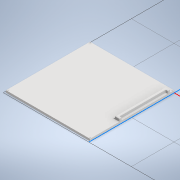
# Autodesk Inventor part: box_bottom
Saved by Autodesk Inventor 2020 (Build 240168000, 168)
## iProperties
Created: 2020-02-22
Part Number: box_bottom
Material: Generic
Document SubType Name: Modeling
Designer: Luka
Density: 1 g/cm^3
Appearance: Default
Author: Luka
Autodesk Inventor part; units mm, degrees
ref_plane "YZ Plane" through (0, 0, 0) normal (1, 0, 0) x (0, 1, 0)
sketch "Sketch1" plane through (0, 0, 0) normal (0, 1, 0) x (-1, 0, 0)
  line L0 (200, 200) -> (0, 200)
  line L1 (0, 200) -> (0, 0)
  line L2 (0, 0) -> (200, 0)
  line L3 (200, 0) -> (200, 200)
  dimension "d0" = 200
  dimension "d1" = 200
  constraints: 8 end point, 2 parallel, 1 horizontal, 1 perpendicular
  measures "d0" distance of L2.end L1.end
  measures "d1" distance of L1.end L0.end
extrude "Extrusion1" add sketch "Sketch1" along normal blind 200
shell "Shell1" thickness 5 removed faces 1 at (-66.6667, 200, 133.3333)
sketch "Sketch2" plane through (-200, 0, 200) normal (0, 0, 1) x (1, 0, 0)
  line L0 (155, 160) -> (158.5, 160)
  line L1 (158.5, 160) -> (158.5, 130)
  line L2 (158.5, 130) -> (155, 130)
  line L3 (155, 130) -> (155, 160)
  line L4 (0, 0) -> (0, 200) projected
  line L5 (200, 0) -> (200, 200) projected
  line L6 (0, 200) -> (200, 200) projected
  line L7 (120, 160) -> (40, 160)
  line L8 (40, 160) -> (40, 125)
  line L9 (40, 125) -> (120, 125)
  line L10 (120, 125) -> (120, 160)
  line L11 (40, 115) -> (120, 115)
  line L12 (120, 115) -> (120, 35)
  line L13 (120, 35) -> (40, 35)
  line L14 (40, 35) -> (40, 115)
  line L15 (69, 25) -> (91, 25)
  line L16 (91, 25) -> (91, 21)
  line L17 (91, 21) -> (69, 21)
  line L18 (69, 21) -> (69, 25)
  line L19 (44, 155) -> (116, 155)
  line L20 (116, 155) -> (116, 130)
  line L21 (116, 130) -> (44, 130)
  line L22 (44, 130) -> (44, 155)
  circle A0 centre (40, 160) radius 5
  circle A1 centre (120, 160) radius 5
  circle A2 centre (120, 125) radius 5
  circle A3 centre (40, 125) radius 5
  line L23 (69, 25) -> (91, 25)
  line L24 (91, 25) -> (91, 35)
  line L25 (91, 35) -> (69, 35)
  line L26 (69, 35) -> (69, 25)
  point P0 (120, 155)
  point P1 (115, 160)
  point P2 (115, 125)
  point P3 (120, 130)
  point P4 (40, 130)
  point P5 (45, 125)
  point P6 (45, 160)
  point P7 (40, 155)
  point P8 (69, 35)
  point P9 (91, 25)
  dimension "COINw" = 3.5
  dimension "COINh" = 30
  dimension "d7" = 155
  dimension "d8" = 41.5
  dimension "d12" = 40
  dimension "d13" = 40
  dimension "LCDw" = 80
  dimension "LCDh" = 35
  dimension "d19" = 22
  dimension "d20" = 4
  dimension "d22" = 29
  dimension "d23" = 10
  dimension "d24" = 10
  dimension "d27" = 72
  dimension "d28" = 25
  dimension "d29" = 4
  dimension "d30" = 4
  dimension "d31" = 5
  dimension "d32" = 5
  dimension "d33" = 10
  dimension "d34" = 10
  dimension "d35" = 10
  constraints: 48 end point, 12 parallel, 7 perpendicular, 6 horizontal, 4 centre point, 4 coincident, 4 collinear, 1 point on line
  measures "COINw" distance of L1.end L2.end
  measures "COINh" distance of L0.end L1.end
  measures "d7" distance between parallel lines of L4 L3
  measures "d8" distance between parallel lines of L5 L1
  measures "d12" distance between parallel lines of L6 L0
  measures "d13" distance between parallel lines of L8 L4
  measures "LCDw" distance between parallel lines of L10 L8
  measures "LCDh" distance between parallel lines of L9 L7
  measures "d19" distance of L15.start L15.end
  measures "d20" distance of L15.end L16.end
  measures "d22" distance from line of L13.end L18
  measures "d23" distance between parallel lines of L15 L13
  measures "d24" distance between parallel lines of L11 L9
  measures "d27" distance of L20.end L21.end
  measures "d28" distance of L19.end L20.end
  measures "d29" distance between parallel lines of L8 L22
  measures "d30" distance between parallel lines of L10 L20
  measures "d31" distance between parallel lines of L7 L19
  measures "d32" distance between parallel lines of L9 L21
  measures "d33" diameter of A0
  measures "d34" diameter of A2
  measures "d35" diameter of A3
extrude "Extrusion2" cut sketch "Sketch2" along normal mid plane 10 contours L0 L1 L2 L3 | L15 L16 L17 L18 | L19 L20 L21 L22
fillet "Fillet1" radius 2 4 edges at (-195, 200, 100) (-100, 200, 5) (-5, 200, 100) (-100, 200, 195)
sketch "Sketch3" plane through (0, 0, 200) normal (1, 0, 0) x (0, 0, -1)
  line L0 (0, 0) -> (0, 200) projected
  line L1 (0, 80) -> (200, 80)
  line L2 (0, 0) -> (200, 0) projected
  line L3 (195, 5) -> (195, 198) projected
  line L4 (195, 80) -> (195, 0)
  line L5 (95, 80) -> (95, 0)
  line L6 (200, 0) -> (0, 0) projected
  line L7 (5, 5) -> (195, 5) projected
  line L8 (95, 5) -> (195, 5)
  dimension "d16" = 80
  dimension "d44" = 100
  constraints: 8 end point, 8 point on line, 2 perpendicular, 1 collinear, 1 horizontal
  measures "d16" distance between parallel lines of L2 L1
  measures "d44" distance between parallel lines of L3 L5
extrude "Extrusion3" cut sketch "Sketch2" against normal blind 2 contours A0 L8 L7 | L7 L8 A0 | L7 A1 L10 A2 L9 A3 L8 A0 | A1 L10 L7 | L7 L10 A1 | A3 L9 L8 | L8 L9 A3 | A2 L9 L10 | L10 L9 A2 | L11 L12 L13 L14 | L13 L24 L15 L26 | L19 L20 L21 L22
hole "Hole1" at (-160, 160, 200) at (-80, 160, 200) at (-80, 125, 200) at (-160, 125, 200) direction (0, 0, -1) diameter 3.5 depth 5
fillet "Fillet2" radius 3 5 edges at (-160, 75, 198) (-80, 75, 198) (-94.5, 35, 198) (-145.5, 35, 198) (-120, 115, 198)
extrude "Extrusion4" cut sketch "Sketch3" against normal blind 5 contours L1 L3 L7 L5
sketch "Sketch4" plane through (0, 5, 105) normal (0, 0, -1) x (-1, 0, 0)
  circle A0 centre (2.5, 73.5) radius 2.5
  line L0 (0, 0) -> (0, 75) projected
  line L1 (5, 75) -> (5, 0) projected
  circle A1 centre (2.5, 73.5) radius 1
  line L2 (0, 75) -> (5, 75) projected
  line L3 (2.5, 76) -> (2.5, 73.5)
  line L4 (2.5, 73.5) -> (2.5, 71)
  line L5 (2.5, 71) -> (5, 71)
  line L6 (2.5, 76) -> (5, 76)
  line L7 (0, 75) -> (5, 75) projected
  line L8 (5, 76) -> (5, 75)
  point P0 (0, -5)
  point P1 (4.5, 75)
  point P2 (0.5, 75)
  dimension "d47" = 2
  dimension "d48" = 1.5
  constraints: 10 end point, 4 tangent, 2 centre point, 2 perpendicular, 2 point on circle, 2 point on line, 1 coincident, 1 parallel, 1 vertical
  measures "d47" diameter of A1
  measures "d48" distance from line of A0.centre L2
extrude "Extrusion5" add sketch "Sketch4" along normal blind 80 contours L4 A1 L3 L2 A0 | A0 L2 L3 A1 L4
extrude "Extrusion6" cut sketch "Sketch4" along normal blind 60 contours L4 A1 L3 L2 A0 | A0 L2 L3 A1 L4
extrude "Extrusion7" add sketch "Sketch4" along normal blind 40 contours L4 A1 L3 L2 A0 | A0 L2 L3 A1 L4
extrude "Extrusion8" cut sketch "Sketch4" along normal blind 20 contours L4 A1 L3 L2 A0 | A0 L2 L3 A1 L4
fillet "Fillet3" radius 3 2 edges at (-0.5, 80, 75) (-0.5, 80, 35)
fillet "Fillet4" radius 4 2 edges at (-4.5, 80, 75) (-4.5, 80, 35)
extrude "Extrusion9" cut sketch "Sketch4" against normal blind 40 contours L4 L3 A1 | A1 L3 L4
ref_plane "Work Plane1" through (0, 5, 120) normal (0, 0, -1) x (-1, 0, 0)
sketch "Sketch5" plane through (0, 5, 120) normal (0, 0, -1) x (-1, 0, 0)
  circle A0 centre (2.5, 73.5) radius 2.5 projected
  circle A1 centre (2.5, 73.5) radius 1 projected
  line L0 (2.5, 71) -> (5, 71) projected
  line L1 (5, 75) -> (5, 0) projected
  line L2 (5, 71) -> (5, 75)
  line L3 (5, 75) -> (5, 76)
  line L4 (5, 75) -> (5, 193) projected
  line L5 (2.5, 76) -> (5, 76)
  line L6 (2.5, 76) -> (2.5, 71)
  point P0 (0, -5)
  constraints: 8 end point, 1 collinear, 1 point on circle, 1 point on line, 1 tangent, 1 vertical
extrude "Extrusion10" cut sketch "Sketch5" against normal blind 25 contours A0 L6 A1 | L1 L0 A0 | A0 L5 L3 L1 | A1 L6 picked at (4.2027, 74.5258) picked at (3.0499, 73.7078)
ref_plane "Work Plane4" through (-195, 5, 5) normal (0, 1, 0) x (1, 0, 0)
split "Split1" plane through (-195, 5, 5) removes the side toward (0, 1, 0)
sketch "Sketch6" plane through (-200, 5, 0) normal (0, 1, 0) x (1, 0, 0)
  line L0 (200, 0) -> (200, -200) projected
  line L1 (200, -10) -> (195, -10)
  line L2 (195, -10) -> (195, -15)
  line L3 (195, -15) -> (200, -15)
  line L4 (0, 0) -> (200, 0) projected
  line L5 (200, -125) -> (195, -125)
  line L6 (195, -125) -> (195, -130)
  line L7 (195, -130) -> (200, -130)
  line L8 (195, -130) -> (190, -130)
  line L9 (190, -130) -> (190, -10)
  line L10 (190, -10) -> (195, -10)
  line L11 (195, -10) -> (195, -130)
  dimension "d66" = 10
  dimension "d67" = 5
  dimension "d68" = 5
  dimension "d71" = 5
  dimension "d72" = 110
  dimension "d73" = 5
  dimension "d89" = 5
  constraints: 20 end point, 5 perpendicular, 4 point on line, 3 horizontal, 2 parallel, 1 collinear
  measures "d66" distance between parallel lines of L4 L1
  measures "d67" distance between parallel lines of L1 L3
  measures "d68" distance between parallel lines of L0 L2
  measures "d71" distance between parallel lines of L0 L6
  measures "d72" distance between parallel lines of L3 L5
  measures "d73" distance between parallel lines of L7 L5
  measures "d89" distance between parallel lines of L9 L11
extrude "Extrusion11" add sketch "Sketch6" along normal blind 6 contours L0 L3 L2 L1 | L2 L11 L6 L8 L9 L10 | L0 L7 L6 L5
sketch "Sketch7" plane through (0, 0, 0) normal (0, -1, 0) x (1, 0, 0)
  line L0 (-200, 200) -> (0, 200) projected
  line L1 (0, 200) -> (0, 0) projected
  line L2 (0, 0) -> (-200, 0) projected
  line L3 (-200, 0) -> (-200, 200) projected
  point P0 (-2.5, 197.5)
  point P1 (-2.5, 2.5)
  point P2 (-197.5, 2.5)
  point P3 (-197.5, 197.5)
  dimension "d74" = 2.5
  dimension "d75" = 2.5
  dimension "d76" = 2.5
  dimension "d77" = 2.5
  dimension "d78" = 2.5
  dimension "d79" = 2.5
  dimension "d80" = 2.5
  dimension "d81" = 2.5
  measures "d74" distance from line of L0 point (-2.5, 197.5)
  measures "d75" distance from line of L1 point (-2.5, 197.5)
  measures "d76" distance from line of L1 point (-2.5, 2.5)
  measures "d77" distance from line of L2 point (-2.5, 2.5)
  measures "d78" distance from line of L0 point (-197.5, 197.5)
  measures "d79" distance from line of L3 point (-197.5, 197.5)
  measures "d80" distance from line of L3 point (-197.5, 2.5)
  measures "d81" distance from line of L2 point (-197.5, 2.5)
hole "Hole2" at (-2.5, 0, 197.5) at (-2.5, 0, 2.5) at (-197.5, 0, 2.5) at (-197.5, 0, 197.5) direction (0, 1, 0) diameter 2 depth 5 counterbore diameter 4 counterbore depth 3
fillet "Fillet5" radius 6 1 edges at (-10, 5, 70)
equation "\"d45\" = SHELLw"
equation "\"SHELLw\" = 5"
body "Solid1"
